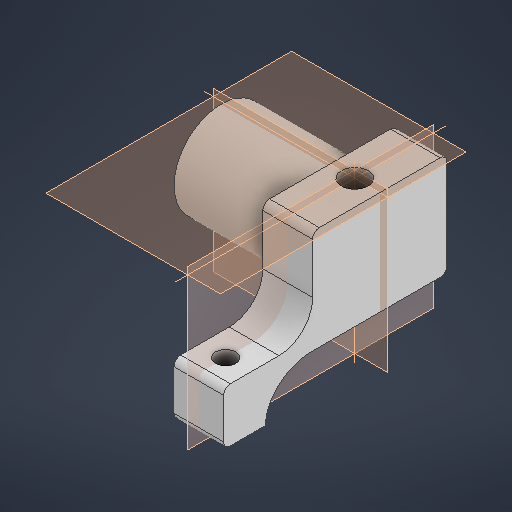
# Autodesk Inventor part: support_avant
Saved by Autodesk Inventor 2027.1 (Build 311270010, 270A)
## iProperties
Created: 2026-09-16
Part Number: support_avant
Material: Generic
Document SubType Name: Modeling
Designer: thiag
Density: 1 g/cm^3
Appearance: Default
Author: thiag
Autodesk Inventor part; units mm, degrees
sketch "Sketch5" plane through (0, 0, 0) normal (1, 0, 0) x (0, 1, 0)
  line L0 (-8.5, 10) -> (0, 10)
  line L1 (0, 10) -> (0, -10)
  line L2 (0, -10) -> (-14.4, -10)
  line L3 (-15.4, -9) -> (-15.4, 10)
  line L4 (-26.0485, 0) -> (4.3414, 0) projected
  line L5 (0, -16.9345) -> (0, 30.1575) projected
  line L6 (-14.5, 23.223) -> (-20.5, 23.223)
  line L7 (-21.5, 22.223) -> (-21.5, 17)
  ellipse E0 centre (-21.5, 10) end of major axis (-21.5, 17) minor radius 6.1 (-15.4, 10) -> (-21.5, 17) ccw
  line L8 (-13.5, 22.223) -> (-13.5, 15)
  arc A0 (-20.5, 23.223) -> (-21.5, 22.223) centre (-20.5, 22.223) ccw
  arc A1 (-13.5, 22.223) -> (-14.5, 23.223) centre (-14.5, 22.223) ccw
  arc A2 (-15.4, -9) -> (-14.4, -10) centre (-14.4, -9) ccw
  arc A3 (-13.5, 15) -> (-8.5, 10) centre (-8.5, 15) ccw
  point P0 (0, 0)
  point P1 (-15.4, -10)
  point P2 (-13.5, 10)
  dimension "d64" = 6.1
  dimension "d78" = 7
  dimension "d31" = 15.4
  dimension "d32" = 20
  dimension "d33" = 10
  dimension "d34" = 15.4
  dimension "d58" = 21.5
  dimension "d59" = 23.223
  dimension "d71" = 8
  dimension "d74" = 1
  dimension "d75" = 1
  dimension "d76" = 0
  dimension "d77" = 5
  constraints: 14 end point, 8 point on circle, 8 tangent, 4 centre point, 4 point on line, 2 horizontal, 2 parallel, 2 perpendicular, 1 equal radius, 4 other
  measures "d31" distance of L1.end point (-15.4, -10)
  measures "d32" distance between parallel lines of L2 L0
  measures "d33" distance between parallel lines of L4 L0
  measures "d34" distance between parallel lines of L5 L3
  measures "d58" distance between parallel lines of L5 L7
  measures "d59" distance between parallel lines of L4 L6
  measures "d71" distance between parallel lines of L8 L7
  measures "d74" radius of A0
  measures "d75" radius of A2
  measures "d76" distance from line of point (-13.5, 10) L0
  measures "d77" radius of A3
extrude "Extrusion4" add sketch "Sketch5" along normal mid plane 7.4
sketch "Sketch6" plane through (-3.7, -15.4, -10) normal (0, -1, 0) x (1, 0, 0)
  circle A0 centre (3.7, 10) radius 2
  line L0 (3.7, 39.8676) -> (3.7, -6.6446) projected
  point P0 (3.7, 10)
  dimension "d37" = 4
  constraints: 1 centre point, 1 coincident
  measures "d37" diameter of A0
extrude "Extrusion5" cut sketch "Sketch6" against normal blind 15.5
sketch "Sketch7" plane through (-3.7, 0, 0) normal (-1, 0, 0) x (0, 0, 1)
  circle A0 centre (0, -7.4) radius 7
  line L0 (10, 0) -> (-10, 0) projected
  line L1 (0, -25.8) -> (0, 4.3) projected
  circle A1 centre (0, -7.4) radius 4
  point P0 (0, 0)
  dimension "d40" = 14
  dimension "d41" = 7.4
  dimension "d42" = 0
  dimension "d43" = 8
  constraints: 2 centre point, 1 coincident
  measures "d40" diameter of A0
  measures "d41" distance from line of L0 A0.centre
  measures "d42" distance from line of L1 A0.centre
  measures "d43" diameter of A1
extrude "Extrusion6" add sketch "Sketch7" along normal blind 16.2 contours A0 L1 A1 | L1 A1 A0
sketch "Sketch8" plane through (-19.9, -7.4, 0) normal (-1, 0, 0) x (0, 0, 1)
  circle A0 centre (0, 0) radius 6.5
  line L0 (0, 11.7) -> (0, -18.4) projected
  line L1 (10, 7.4) -> (-10, 7.4) projected
  point P0 (0, 7.4)
  dimension "d46" = 13
  dimension "d47" = 0
  dimension "d48" = 7.4
  constraints: 1 centre point
  measures "d46" diameter of A0
  measures "d47" distance from line of L0 A0.centre
  measures "d48" distance from line of L1 A0.centre
extrude "Extrusion7" cut sketch "Sketch8" against normal blind 12.3
sketch "Sketch10" plane through (-3.7, -21.5, 17) normal (0, -1, 0) x (1, 0, 0)
  circle A0 centre (3.7, 2.223) radius 1.5
  line L0 (-1.48, -17) -> (8.88, -17) projected
  line L1 (3.7, 12.8676) -> (3.7, -33.6446) projected
  point P0 (3.7, -17)
  dimension "d82" = 3
  dimension "d83" = 19.223
  dimension "d84" = 0
  constraints: 1 centre point
  measures "d82" diameter of A0
  measures "d83" distance from line of L0 A0.centre
  measures "d84" distance from line of L1 A0.centre
extrude "Extrusion8" cut sketch "Sketch10" against normal blind 8
fillet "Fillet1" radius 1 1 edges at (0, 0, -10)
fillet "Fillet2" radius 1 1 edges at (0, 0, 10)
body "Solid2"
